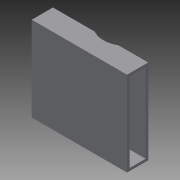
# Autodesk Inventor part: Front Fender BoxBeam
Saved by Autodesk Inventor 2015 (Build 190159000, 159)
## iProperties
Created: 2015-02-14
Part Number: Front Fender BoxBeam
Material: Generic
Document SubType Name: Modeling
Designer: chapale16
Density: 1 g/cm^3
Appearance: Default
Author: chapale16
Autodesk Inventor part; units mm, degrees
ref_plane "YZ Plane" through (0, 0, 0) normal (1, 0, 0) x (0, 1, 0)
ref_plane "XZ Plane" through (0, 0, 0) normal (0, 1, 0) x (-1, 0, 0)
ref_plane "XY Plane" through (0, 0, 0) normal (0, 0, 1) x (1, 0, 0)
sketch "Sketch1" plane through (0, 0, 0) normal (1, 0, 0) x (0, 1, 0)
  line L0 (0, 0) -> (-101.6, 0)
  line L1 (-101.6, 0) -> (-101.6, -25.4)
  line L2 (-101.6, -25.4) -> (0, -25.4)
  line L3 (0, -25.4) -> (0, 0)
  line L4 (-3.175, -22.225) -> (-98.425, -22.225)
  line L5 (-98.425, -22.225) -> (-98.425, -3.175)
  line L6 (-98.425, -3.175) -> (-3.175, -3.175)
  line L7 (-3.175, -3.175) -> (-3.175, -22.225)
  dimension "d0" = 101.6
  dimension "d1" = 25.4
  dimension "d2" = 3.175
  constraints: 16 end point, 4 parallel, 2 perpendicular, 1 horizontal, 3 other
  measures "d0" distance of L2.end L1.end
  measures "d1" distance of L1.end L0.end
  measures "d2" distance between parallel lines of L2 L4
extrude "Extrusion1" add sketch "Sketch1" along normal blind 114.3
sketch "Sketch2" plane through (0, 0, 0) normal (0, 1, 0) x (1, 0, 0)
  line L0 (0, 25.4) -> (0, 0) projected
  line L1 (0, 0) -> (114.3, 0) projected
  line L2 (114.3, 25.4) -> (114.3, 0) projected
  line L3 (0, 25.4) -> (114.3, 25.4) projected
  circle A0 centre (64.3357, 49.9643) radius 6.35 projected
  circle A1 centre (64.3357, 49.9643) radius 28.3845 projected
extrude "Extrusion2" cut sketch "Sketch2" against normal blind 114.3 contours A1 L3 | L3 A1
sketch "Sketch3" plane through (0, 0, 0) normal (0, 1, 0) x (1, 0, 0)
  circle A0 centre (23.3357, 12.7) radius 3.175 projected
  circle A1 centre (105.3357, 12.7) radius 3.175 projected
  point P0 (0, 0)
extrude "Extrusion3" cut sketch "Sketch3" against normal blind 12.7
sketch "Sketch4" plane through (0, -101.6, 0) normal (0, 0, 1) x (1, 0, 0)
  point P0 (0, 101.6)
  point P1 (55.5752, 14.3002)
  point P2 (55.5752, 39.7002)
hole "Hole1" at (55.5752, -87.2998, 0) at (55.5752, -61.8998, 0) direction (0, 0, -1) diameter 6.35 end through all
body "Solid1"
